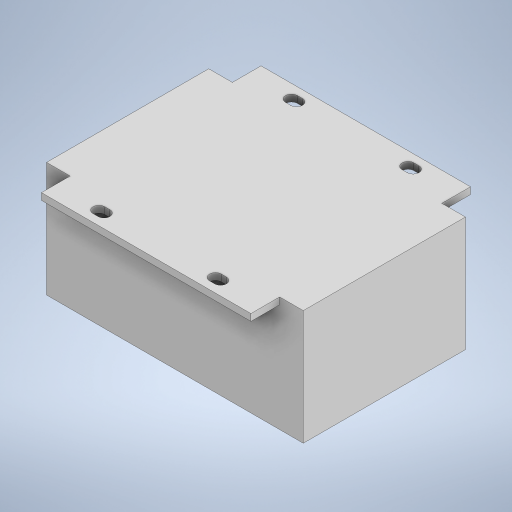
# Autodesk Inventor part: N0039 ERAM-0.01-1G-2W
Saved by Autodesk Inventor 2023 (Build 270158000, 158)
## iProperties
Created: 2023-10-03
Part Number: N0039 ERAM-0.01-1G-2W
Material: 一般
Document SubType Name: Modeling
Designer: 310611102
Density: 1 g/cm^3
Appearance: 預設
Author: 310611102
Autodesk Inventor part; units mm, degrees
ref_plane "YZ Plane" through (0, 0, 0) normal (1, 0, 0) x (0, 1, 0)
ref_plane "XZ Plane" through (0, 0, 0) normal (0, 1, 0) x (-1, 0, 0)
ref_plane "XY Plane" through (0, 0, 0) normal (0, 0, 1) x (1, 0, 0)
sketch "Sketch1" plane through (0, 0, 0) normal (0, 0, 1) x (1, 0, 0)
  line L0 (-38, 16) -> (38, 16)
  line L1 (38, 16) -> (38, -16)
  line L2 (38, -16) -> (-38, -16)
  line L3 (-38, -16) -> (-38, 16)
  line L4 (-38, 16) -> (38, -16) construction
  line L5 (38, 16) -> (-38, -16) construction
  point P0 (0, 0)
  dimension "d0" = 76
  dimension "d1" = 32
  constraints: 12 end point, 2 midpoint, 2 parallel, 1 horizontal, 1 perpendicular
  measures "d0" distance of L0.start L0.end
  measures "d1" distance of L0.end L1.end
extrude "Extrusion1" add sketch "Sketch1" along normal mid plane 48
sketch "Sketch2" plane through (-38, 16, 24) normal (0, 1, 0) x (1, 0, 0)
  line L0 (69, -8.5) -> (7, -8.5)
  line L1 (7, -8.5) -> (7, 56.5)
  line L2 (7, 56.5) -> (69, 56.5)
  line L3 (69, 56.5) -> (69, -8.5)
  line L4 (69, -8.5) -> (7, 56.5) construction
  line L5 (7, -8.5) -> (69, 56.5) construction
  line L6 (7, 48) -> (0, 48)
  line L7 (0, 48) -> (0, 0)
  line L8 (0, 0) -> (7, 0)
  line L9 (7, 0) -> (7, 48)
  line L10 (7, 48) -> (0, 0) construction
  line L11 (0, 48) -> (7, 0) construction
  line L12 (76, 48) -> (69, 48)
  line L13 (69, 48) -> (69, 0)
  line L14 (69, 0) -> (76, 0)
  line L15 (76, 0) -> (76, 48)
  line L16 (76, 48) -> (69, 0) construction
  line L17 (69, 48) -> (76, 0) construction
  line L18 (0, 48) -> (76, 48) projected
  line L19 (76, 48) -> (76, 0) projected
  line L20 (20, -4.5) -> (21.5, -4.5) construction
  line L21 (20, -6.25) -> (21.5, -6.25)
  line L22 (21.5, -2.75) -> (20, -2.75)
  arc A0 (20, -2.75) -> (20, -6.25) centre (20, -4.5) ccw
  arc A1 (21.5, -6.25) -> (21.5, -2.75) centre (21.5, -4.5) ccw
  line L23 (28.4806, 24) -> (38, 24) construction
  line L24 (38, 24) -> (38, 34.5741) construction
  line L25 (20, 52.5) -> (21.5, 52.5) construction
  line L26 (20, 54.25) -> (21.5, 54.25)
  line L27 (21.5, 50.75) -> (20, 50.75)
  arc A2 (20, 54.25) -> (20, 50.75) centre (20, 52.5) ccw
  arc A3 (21.5, 50.75) -> (21.5, 54.25) centre (21.5, 52.5) ccw
  line L28 (56, -4.5) -> (54.5, -4.5) construction
  line L29 (56, -6.25) -> (54.5, -6.25)
  line L30 (54.5, -2.75) -> (56, -2.75)
  arc A4 (56, -6.25) -> (56, -2.75) centre (56, -4.5) ccw
  arc A5 (54.5, -2.75) -> (54.5, -6.25) centre (54.5, -4.5) ccw
  line L31 (56, 54.25) -> (54.5, 54.25)
  line L32 (56, 52.5) -> (54.5, 52.5) construction
  line L33 (54.5, 50.75) -> (56, 50.75)
  arc A6 (54.5, 54.25) -> (54.5, 50.75) centre (54.5, 52.5) ccw
  arc A7 (56, 50.75) -> (56, 54.25) centre (56, 52.5) ccw
  point P0 (3.5, 24)
  point P1 (72.5, 24)
  point P2 (20.75, -4.5)
  point P3 (20.75, 52.5)
  point P4 (55.25, -4.5)
  point P5 (55.25, 52.5)
  point P6 (23.25, -4.5)
  point P7 (18.25, -4.5)
  point P8 (20.75, -6.25)
  point P9 (20.75, -2.75)
  point P10 (20.75, 52.5)
  point P11 (55.25, -4.5)
  point P12 (69, 48)
  point P13 (7, 48)
  point P14 (7, 0)
  dimension "d4" = 65
  dimension "d5" = 62
  dimension "d6" = 5
  dimension "d7" = 3.5
  dimension "d8" = 57
  dimension "d12" = 36
  constraints: 72 end point, 21 symmetric about line, 18 point on circle, 11 midpoint, 8 centre point, 7 parallel, 5 horizontal, 4 tangent, 3 collinear, 3 perpendicular, 2 point on line, 1 vertical, 6 other
  measures "d4" distance between parallel lines of L0 L2
  measures "d5" distance of L1.end L2.end
  measures "d6" distance of point (23.25, -4.5) point (18.25, -4.5)
  measures "d7" distance of point (20.75, -6.25) point (20.75, -2.75)
  measures "d8" distance of point (20.75, 52.5) point (20.75, -4.5)
  measures "d12" distance of L28.start L20.start
extrude "Extrusion2" add sketch "Sketch2" along normal blind 2
body "Solid1"
